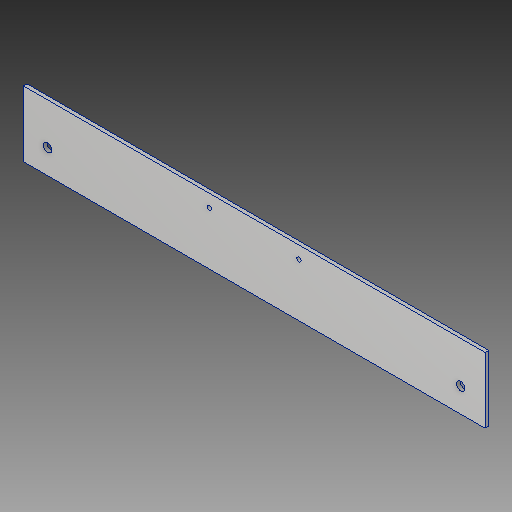
# Autodesk Inventor part: SupportsheetMonitor
Saved by Autodesk Inventor 2017 (Build 210142000, 142)
## iProperties
Created: 2016-11-08
Part Number: SupportsheetMonitor
Material: Aluminum 6061
Document SubType Name: Modeling
Designer: Jonis
Density: 2.7 g/cm^3
Appearance: Aluminum - Flat
Author: Jonis
Autodesk Inventor part; units mm, degrees
ref_plane "YZ Plane" through (0, 0, 0) normal (1, 0, 0) x (0, 1, 0)
ref_plane "XZ Plane" through (0, 0, 0) normal (0, 1, 0) x (-1, 0, 0)
ref_plane "XY Plane" through (0, 0, 0) normal (0, 0, 1) x (1, 0, 0)
sketch "Sketch1" plane through (0, 0, 0) normal (0, 0, 1) x (1, 0, 0)
  line L0 (0, 0) -> (380, 0)
  line L1 (380, 0) -> (380, 54)
  line L2 (380, 54) -> (0, 54)
  line L3 (0, 54) -> (0, 0)
  dimension "d0" = 380
  dimension "d1" = 54
  constraints: 8 end point, 2 parallel, 1 horizontal, 1 perpendicular
  measures "d0" distance of L2.end L1.end
  measures "d1" distance of L1.end L0.end
extrude "Extrusion1" add sketch "Sketch1" along normal blind 3
sketch "Sketch2" plane through (0, 0, 3) normal (0, 0, 1) x (1, 0, 0)
  line L0 (0, 54) -> (0, 0) projected
  line L1 (380, 54) -> (0, 54) projected
  line L2 (0, 0) -> (380, 0) projected
  line L3 (380, 0) -> (380, 54) projected
  point P0 (20, 20)
  point P1 (360, 20)
  dimension "d4" = 20
  dimension "d6" = 20
  dimension "d7" = 20
  dimension "d8" = 20
  measures "d4" distance from line of L0 point (20, 20)
  measures "d6" distance from line of L2 point (20, 20)
  measures "d7" distance from line of L2 point (360, 20)
  measures "d8" distance from line of L3 point (360, 20)
hole "Hole1" at (20, 20, 3) at (360, 20, 3) direction (0, 0, -1) diameter 7 end through all
sketch "Sketch3" plane through (0, 0, 3) normal (0, 0, 1) x (1, 0, 0)
  line L0 (0, 54) -> (0, 0) projected
  line L1 (380, 54) -> (0, 54) projected
  point P0 (153.17, 43.69)
  point P1 (226.83, 43.69)
  dimension "d16" = 73.66
  dimension "d17" = 153.17
  dimension "d18" = 10.31
  dimension "d19" = 10.31
  measures "d16" distance of point (226.83, 43.69) point (153.17, 43.69)
  measures "d17" distance from line of L0 point (153.17, 43.69)
  measures "d18" distance from line of L1 point (153.17, 43.69)
  measures "d19" distance from line of L1 point (226.83, 43.69)
hole "Hole2" at (153.17, 43.69, 3) at (226.83, 43.69, 3) direction (0, 0, -1) diameter 3.5 end through all
body "Solid1"
